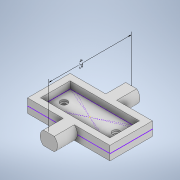
# Autodesk Inventor part: connectorToTubeBracketWithHexShaft
Saved by Autodesk Inventor 2021.1 (Build 251245010, 245A)
## iProperties
Created: 2020-07-21
Part Number: connectorToTubeBracketWithHexShaft
Material: Generic
Document SubType Name: Modeling
Designer: robst
Density: 1 g/cm^3
Appearance: Default
Author: robst
Autodesk Inventor part; units mm, degrees
ref_plane "YZ Plane" through (0, 0, 0) normal (1, 0, 0) x (0, 1, 0)
ref_plane "XZ Plane" through (0, 0, 0) normal (0, 1, 0) x (-1, 0, 0)
ref_plane "XY Plane" through (0, 0, 0) normal (0, 0, 1) x (1, 0, 0)
sketch "Sketch1" plane through (0, 0, 0) normal (0, 1, 0) x (-1, 0, 0)
  line L0 (50.8, 21.59) -> (-50.8, 21.59)
  line L1 (-50.8, 21.59) -> (-50.8, -21.59)
  line L2 (-50.8, -21.59) -> (50.8, -21.59)
  line L3 (50.8, -21.59) -> (50.8, 21.59)
  line L4 (50.8, 21.59) -> (-50.8, -21.59) construction
  line L5 (-50.8, 21.59) -> (50.8, -21.59) construction
  line L6 (60.325, 31.115) -> (-60.325, 31.115)
  line L7 (-60.325, 31.115) -> (-60.325, -31.115)
  line L8 (-60.325, -31.115) -> (60.325, -31.115)
  line L9 (60.325, -31.115) -> (60.325, 31.115)
  line L10 (60.325, 31.115) -> (-60.325, -31.115) construction
  line L11 (-60.325, 31.115) -> (60.325, -31.115) construction
  point P0 (0, 0)
  constraints: 24 end point, 4 midpoint, 4 parallel, 2 horizontal, 2 perpendicular
extrude "Extrusion1" add sketch "Sketch1" against normal blind 9.525 contours L3 L2 L1 L0 | L9 L8 L7 L6
extrude "Extrusion2" add sketch "Sketch1" along normal blind 10.16
sketch "Sketch4" plane through (-60.325, -9.525, 31.115) normal (0, 0, 1) x (1, 0, 0)
  line L0 (0, 0) -> (0, 19.685) projected
  line L1 (120.65, 0) -> (0, 0) projected
  line L2 (0, 19.685) -> (120.65, 19.685) projected
  line L3 (9.525, 19.685) -> (111.125, 19.685) projected
  line L4 (52.2991, 19.685) -> (68.3509, 19.685)
  line L5 (0, 0) -> (120.65, 0) projected
  line L6 (52.2991, 0) -> (68.3509, 0)
  arc A0 (52.2991, 19.685) -> (52.2991, 0) centre (60.325, 9.8425) ccw
  arc A1 (68.3509, 0) -> (68.3509, 19.685) centre (60.325, 9.8425) ccw
  point P0 (60.325, 9.525)
  dimension "d10" = 9.8425
  constraints: 4 end point, 4 point on circle, 4 point on line, 2 centre point
  measures "d10" distance from line of A0.centre L1
extrude "Extrusion4" add sketch "Sketch4" along normal blind 29.21 contours A0 L2 A1 L1
mirror "Mirror1" about plane through (0, 0, 0) normal (0, 0, 1) of "Extrusion4"
sketch "Sketch5" plane through (0, 0, 0) normal (0, 1, 0) x (1, 0, 0)
  line L0 (-50.8, 21.59) -> (-50.8, -21.59) projected
  line L1 (50.8, -21.59) -> (50.8, 21.59) projected
  point P0 (0, 0)
  point P1 (-38.1, 0)
  point P2 (38.1, 0)
  dimension "postHoleCenter" = 12.7
  dimension "d16" = 12.7
  measures "postHoleCenter" distance from line of L0 point (-38.1, 0)
  measures "d16" distance from line of L1 point (38.1, 0)
hole "Hole1" at (-38.1, 0, 0) at (38.1, 0, 0) direction (0, -1, 0) diameter 5.1054 end through all counterbore diameter 10.16 counterbore depth 2.54 clearance for "Hex Machine Screw" size "#10" standard "Ansi Unified Screw Threads"
equation "\"d4\" = wallThickness"
equation "\"d10\" = 0.5 * outerHeight"
equation "\"d13\" = -0.5 * outerWidth + 0.5 * overallWidth"
equation "\"d16\" = postHoleCenter"
equation "\"wallThickness\" = 9.525"
equation "\"outerWidth\" = innerWidth + 2 * wallThickness"
equation "\"outerLength\" = innerLength + 2 * wallThickness"
equation "\"outerHeight\" = innerDepth + wallThickness"
equation "\"shortenForTestPrint\" = 76.2"
equation "\"overallWidth\" = 120.65"
equation "\"innerWidth\" = 43.18"
equation "\"innerLength\" = 101.6"
equation "\"innerDepth\" = 10.16"
body "Solid1"
